Autodesk Inventor part; units mm, degrees
(part 2 of 2)
sketch "Sketch2" plane through (-23.709139, -13.853617, 14.249199) normal (0, 0.9970894, 0.0762418) x (1, 0, 0)
  line L0 (0, 0.624975) -> (-23.2, 0.624975)
  line L1 (0, 0.624975) -> (-23.2, 0.624975)
  line L2 (-23.2, 0.624975) -> (-23.2, 65.920816)
  line L3 (-23.2, 65.920816) -> (0, 65.920816)
  line L4 (0, 65.920816) -> (0, 0.624975)
  circle A0 centre (-9.208398, 23.610194) radius 8 construction
  circle A1 centre (-13, 35.626174) radius 9.6 construction
  circle A2 centre (-9.208398, 23.610194) radius 8.4
  circle A3 centre (-13, 35.626174) radius 10
  circle A4 centre (-9.208398, 23.610194) radius 1.25
  arc A5 (-17.179273, 22.928177) -> (-16.018307, 22.666389) centre (-15.506202, 27.642647) ccw
  arc A6 (-16.018307, 22.666389) -> (-15.959579, 22.311279) centre (-9.208398, 23.610194) ccw
  arc A7 (-15.959579, 22.311279) -> (-16.974447, 21.689654) centre (-13.872622, 17.764852) ccw
  arc A8 (-16.974447, 21.689654) -> (-16.863291, 21.285842) centre (-9.208398, 23.610194) ccw
  arc A9 (-16.863291, 21.285842) -> (-15.673266, 21.271154) centre (-16.206974, 26.245141) ccw
  arc A10 (-15.673266, 21.271154) -> (-15.54199, 20.936014) centre (-9.208398, 23.610194) ccw
  arc A11 (-15.54199, 20.936014) -> (-16.405438, 20.11697) centre (-12.555382, 16.92284) ccw
  arc A12 (-16.405438, 20.11697) -> (-16.212753, 19.745093) centre (-9.208398, 23.610194) ccw
  arc A13 (-16.212753, 19.745093) -> (-15.045679, 19.978146) centre (-16.601875, 24.732476) ccw
  arc A14 (-15.045679, 19.978146) -> (-14.847592, 19.677624) centre (-9.208398, 23.610194) ccw
  arc A15 (-14.847592, 19.677624) -> (-15.521883, 18.696957) centre (-11.091863, 16.373097) ccw
  arc A16 (-15.521883, 18.696957) -> (-15.256092, 18.373268) centre (-9.208398, 23.610194) ccw
  arc A17 (-15.256092, 18.373268) -> (-14.162975, 18.843876) centre (-16.673645, 23.170761) ccw
  arc A18 (-14.162975, 18.843876) -> (-13.906735, 18.591106) centre (-9.208398, 23.610194) ccw
  arc A19 (-13.906735, 18.591106) -> (-14.362399, 17.491675) centre (-9.546028, 16.139651) ccw
  arc A20 (-14.362399, 17.491675) -> (-14.035117, 17.230321) centre (-9.208398, 23.610194) ccw
  arc A21 (-14.035117, 17.230321) -> (-13.063732, 17.917917) centre (-16.419148, 21.628251) ccw
  arc A22 (-13.063732, 17.917917) -> (-12.760538, 17.723945) centre (-9.208398, 23.610194) ccw
  arc A23 (-12.760538, 17.723945) -> (-12.97766, 16.553803) centre (-7.985437, 16.232703) ccw
  arc A24 (-12.97766, 16.553803) -> (-12.603191, 16.366205) centre (-9.208398, 23.610194) ccw
  arc A25 (-12.603191, 16.366205) -> (-11.795993, 17.240738) centre (-15.849507, 20.172362) ccw
  arc A26 (-11.795993, 17.240738) -> (-11.459095, 17.114043) centre (-9.208398, 23.610194) ccw
  arc A27 (-11.459095, 17.114043) -> (-11.428186, 15.924328) centre (-6.478294, 16.648187) ccw
  arc A28 (-11.428186, 15.924328) -> (-11.022897, 15.818687) centre (-9.208398, 23.610194) ccw
  arc A29 (-11.022897, 15.818687) -> (-10.415163, 16.841935) centre (-14.989617, 18.866723) ccw
  arc A30 (-10.415163, 16.841935) -> (-10.059286, 16.788053) centre (-9.208398, 23.610194) ccw
  arc A31 (-10.059286, 16.788053) -> (-9.781697, 15.630763) centre (-5.090471, 17.367944) ccw
  arc A32 (-9.781697, 15.630763) -> (-9.3633, 15.611694) centre (-9.208398, 23.610194) ccw
  arc A33 (-9.3633, 15.611694) -> (-8.981592, 16.738937) centre (-13.87706, 17.768396) ccw
  arc A34 (-8.981592, 16.738937) -> (-8.622289, 16.760224) centre (-9.208398, 23.610194) ccw
  arc A35 (-8.622289, 16.760224) -> (-8.110152, 15.685937) centre (-3.882621, 18.360517) ccw
  arc A36 (-8.110152, 15.685937) -> (-7.696933, 15.754275) centre (-9.208398, 23.610194) ccw
  arc A37 (-7.696933, 15.754275) -> (-7.557934, 16.936246) centre (-12.560461, 16.925384) ccw
  arc A38 (-7.557934, 16.936246) -> (-7.210908, 17.031771) centre (-9.208398, 23.610194) ccw
  arc A39 (-7.210908, 17.031771) -> (-6.486605, 16.087439) centre (-2.907532, 19.582526) ccw
  arc A40 (-6.486605, 16.087439) -> (-6.096625, 16.240197) centre (-9.208398, 23.610194) ccw
  arc A41 (-6.096625, 16.240197) -> (-6.206408, 17.425238) centre (-11.09736, 16.37453) ccw
  arc A42 (-6.206408, 17.425238) -> (-5.886827, 17.590827) centre (-9.208398, 23.610194) ccw
  arc A43 (-5.886827, 17.590827) -> (-4.982014, 16.817722) centre (-2.207822, 20.980564) ccw
  arc A44 (-4.982014, 16.817722) -> (-4.632316, 17.048223) centre (-9.208398, 23.610194) ccw
  arc A45 (-4.632316, 17.048223) -> (-4.986084, 18.184543) centre (-9.551702, 16.139909) ccw
  arc A46 (-4.986084, 18.184543) -> (-4.707914, 18.412958) centre (-9.208398, 23.610194) ccw
  arc A47 (-4.707914, 18.412958) -> (-3.662136, 17.844868) centre (-1.81407, 22.493529) ccw
  arc A48 (-3.662136, 17.844868) -> (-3.368003, 18.143039) centre (-9.208398, 23.610194) ccw
  arc A49 (-3.368003, 18.143039) -> (-3.950295, 19.180975) centre (-7.991041, 16.231776) ccw
  arc A50 (-3.950295, 19.180975) -> (-3.725694, 19.462233) centre (-9.208398, 23.610194) ccw
  arc A51 (-3.725694, 19.462233) -> (-2.584657, 19.123987) centre (-1.743487, 24.055298) ccw
  arc A52 (-2.584657, 19.123987) -> (-2.358945, 19.476795) centre (-9.208398, 23.610194) ccw
  arc A53 (-2.358945, 19.476795) -> (-3.144311, 20.370985) centre (-6.483583, 16.646115) ccw
  arc A54 (-3.144311, 20.370985) -> (-2.983095, 20.692794) centre (-9.208398, 23.610194) ccw
  arc A55 (-2.983095, 20.692794) -> (-1.796667, 20.599175) centre (-1.999155, 25.597614) ccw
  arc A56 (-1.796667, 20.599175) -> (-1.649239, 20.991201) centre (-9.208398, 23.610194) ccw
  arc A57 (-1.649239, 20.991201) -> (-2.603356, 21.702564) centre (-5.095213, 17.364818) ccw
  arc A58 (-2.603356, 21.702564) -> (-2.512571, 22.05086) centre (-9.208398, 23.610194) ccw
  arc A59 (-2.512571, 22.05086) -> (-1.332604, 22.205958) centre (-2.569902, 27.05307) ccw
  arc A60 (-1.332604, 22.205958) -> (-1.269906, 22.62007) centre (-9.208398, 23.610194) ccw
  arc A61 (-1.269906, 22.62007) -> (-2.351074, 23.117516) centre (-3.886609, 18.356473) ccw
  arc A62 (-2.351074, 23.117516) -> (-2.334687, 23.477076) centre (-9.208398, 23.610194) ccw
  arc A63 (-2.334687, 23.477076) -> (-1.212752, 23.874114) centre (-3.430783, 28.358056) ccw
  arc A64 (-1.212752, 23.874114) -> (-1.237523, 24.292212) centre (-9.208398, 23.610194) ccw
  arc A65 (-1.237523, 24.292212) -> (-2.398489, 24.554) centre (-2.910593, 19.577742) ccw
  arc A66 (-2.398489, 24.554) -> (-2.457217, 24.909109) centre (-9.208398, 23.610194) ccw
  arc A67 (-2.457217, 24.909109) -> (-1.442348, 25.530735) centre (-4.544174, 29.455537) ccw
  arc A68 (-1.442348, 25.530735) -> (-1.553505, 25.934546) centre (-9.208398, 23.610194) ccw
  arc A69 (-1.553505, 25.934546) -> (-2.74353, 25.949235) centre (-2.209821, 20.975248) ccw
  arc A70 (-2.74353, 25.949235) -> (-2.874806, 26.284374) centre (-9.208398, 23.610194) ccw
  arc A71 (-2.874806, 26.284374) -> (-2.011358, 27.103419) centre (-5.861413, 30.297549) ccw
  arc A72 (-2.011358, 27.103419) -> (-2.204043, 27.475295) centre (-9.208398, 23.610194) ccw
  arc A73 (-2.204043, 27.475295) -> (-3.371117, 27.242243) centre (-1.814921, 22.487913) ccw
  arc A74 (-3.371117, 27.242243) -> (-3.569203, 27.542765) centre (-9.208398, 23.610194) ccw
  arc A75 (-3.569203, 27.542765) -> (-2.894913, 28.523432) centre (-7.324932, 30.847292) ccw
  arc A76 (-2.894913, 28.523432) -> (-3.160704, 28.847121) centre (-9.208398, 23.610194) ccw
  arc A77 (-3.160704, 28.847121) -> (-4.253821, 28.376513) centre (-1.743151, 24.049628) ccw
  arc A78 (-4.253821, 28.376513) -> (-4.510061, 28.629283) centre (-9.208398, 23.610194) ccw
  arc A79 (-4.510061, 28.629283) -> (-4.054397, 29.728714) centre (-8.870768, 31.080738) ccw
  arc A80 (-4.054397, 29.728714) -> (-4.381679, 29.990068) centre (-9.208398, 23.610194) ccw
  arc A81 (-4.381679, 29.990068) -> (-5.353064, 29.302472) centre (-1.997648, 25.592138) ccw
  arc A82 (-5.353064, 29.302472) -> (-5.656258, 29.496443) centre (-9.208398, 23.610194) ccw
  arc A83 (-5.656258, 29.496443) -> (-5.439136, 30.666586) centre (-10.431359, 30.987686) ccw
  arc A84 (-5.439136, 30.666586) -> (-5.813605, 30.854184) centre (-9.208398, 23.610194) ccw
  arc A85 (-5.813605, 30.854184) -> (-6.620803, 29.979651) centre (-2.567289, 27.048027) ccw
  arc A86 (-6.620803, 29.979651) -> (-6.957701, 30.106346) centre (-9.208398, 23.610194) ccw
  arc A87 (-6.957701, 30.106346) -> (-6.98861, 31.296061) centre (-11.938501, 30.572202) ccw
  arc A88 (-6.98861, 31.296061) -> (-7.393899, 31.401702) centre (-9.208398, 23.610194) ccw
  arc A89 (-7.393899, 31.401702) -> (-8.001633, 30.378454) centre (-3.427179, 28.353666) ccw
  arc A90 (-8.001633, 30.378454) -> (-8.35751, 30.432336) centre (-9.208398, 23.610194) ccw
  arc A91 (-8.35751, 30.432336) -> (-8.635099, 31.589626) centre (-13.326325, 29.852445) ccw
  arc A92 (-8.635099, 31.589626) -> (-9.053496, 31.608695) centre (-9.208398, 23.610194) ccw
  arc A93 (-9.053496, 31.608695) -> (-9.435204, 30.481452) centre (-4.539735, 29.451993) ccw
  arc A94 (-9.435204, 30.481452) -> (-9.794507, 30.460165) centre (-9.208398, 23.610194) ccw
  arc A95 (-9.794507, 30.460165) -> (-10.306644, 31.534452) centre (-14.534175, 28.859872) ccw
  arc A96 (-10.306644, 31.534452) -> (-10.719863, 31.466114) centre (-9.208398, 23.610194) ccw
  arc A97 (-10.719863, 31.466114) -> (-10.858862, 30.284143) centre (-5.856335, 30.295005) ccw
  arc A98 (-10.858862, 30.284143) -> (-11.205888, 30.188618) centre (-9.208398, 23.610194) ccw
  arc A99 (-11.205888, 30.188618) -> (-11.930191, 31.13295) centre (-15.509264, 27.637863) ccw
  arc A100 (-11.930191, 31.13295) -> (-12.320171, 30.980192) centre (-9.208398, 23.610194) ccw
  arc A101 (-12.320171, 30.980192) -> (-12.210388, 29.795151) centre (-7.319436, 30.845859) ccw
  arc A102 (-12.210388, 29.795151) -> (-12.529969, 29.629562) centre (-9.208398, 23.610194) ccw
  arc A103 (-12.529969, 29.629562) -> (-13.434782, 30.402667) centre (-16.208974, 26.239825) ccw
  arc A104 (-13.434782, 30.402667) -> (-13.78448, 30.172166) centre (-9.208398, 23.610194) ccw
  arc A105 (-13.78448, 30.172166) -> (-13.430712, 29.035846) centre (-8.865094, 31.08048) ccw
  arc A106 (-13.430712, 29.035846) -> (-13.708882, 28.807431) centre (-9.208398, 23.610194) ccw
  arc A107 (-13.708882, 28.807431) -> (-14.754659, 29.37552) centre (-16.602725, 24.726859) ccw
  arc A108 (-14.754659, 29.37552) -> (-15.048792, 29.07735) centre (-9.208398, 23.610194) ccw
  arc A109 (-15.048792, 29.07735) -> (-14.4665, 28.039414) centre (-10.425755, 30.988613) ccw
  arc A110 (-14.4665, 28.039414) -> (-14.691102, 27.758156) centre (-9.208398, 23.610194) ccw
  arc A111 (-14.691102, 27.758156) -> (-15.832139, 28.096402) centre (-16.673309, 23.165091) ccw
  arc A112 (-15.832139, 28.096402) -> (-16.057851, 27.743594) centre (-9.208398, 23.610194) ccw
  arc A113 (-16.057851, 27.743594) -> (-15.272485, 26.849404) centre (-11.933213, 30.574274) ccw
  arc A114 (-15.272485, 26.849404) -> (-15.433701, 26.527595) centre (-9.208398, 23.610194) ccw
  arc A115 (-15.433701, 26.527595) -> (-16.620129, 26.621214) centre (-16.417641, 21.622775) ccw
  arc A116 (-16.620129, 26.621214) -> (-16.767556, 26.229187) centre (-9.208398, 23.610194) ccw
  arc A117 (-16.767556, 26.229187) -> (-15.813439, 25.517825) centre (-13.321582, 29.855571) ccw
  arc A118 (-15.813439, 25.517825) -> (-15.904225, 25.169529) centre (-9.208398, 23.610194) ccw
  arc A119 (-15.904225, 25.169529) -> (-17.084191, 25.01443) centre (-15.846894, 20.167319) ccw
  arc A120 (-17.084191, 25.01443) -> (-17.14689, 24.600319) centre (-9.208398, 23.610194) ccw
  arc A121 (-17.14689, 24.600319) -> (-16.065722, 24.102873) centre (-14.530186, 28.863916) ccw
  arc A122 (-16.065722, 24.102873) -> (-16.082109, 23.743313) centre (-9.208398, 23.610194) ccw
  arc A123 (-16.082109, 23.743313) -> (-17.204043, 23.346275) centre (-14.986013, 18.862333) ccw
  arc A124 (-17.204043, 23.346275) -> (-17.179273, 22.928177) centre (-9.208398, 23.610194) ccw
  arc A125 (-20.63224, 38.75849) -> (-22.059739, 38.801252) centre (-21.52446, 32.822118) ccw
  arc A126 (-22.059739, 38.801252) -> (-22.213494, 38.322751) centre (-13, 35.626174) ccw
  arc A127 (-22.213494, 38.322751) -> (-21.028277, 37.525981) centre (-18.295517, 42.87094) ccw
  arc A128 (-21.028277, 37.525981) -> (-21.116703, 37.10321) centre (-13, 35.626174) ccw
  arc A129 (-21.116703, 37.10321) -> (-22.521898, 36.848243) centre (-20.755184, 31.111058) ccw
  arc A130 (-22.521898, 36.848243) -> (-22.572807, 36.348231) centre (-13, 35.626174) ccw
  arc A131 (-22.572807, 36.348231) -> (-21.247832, 35.815293) centre (-19.686069, 41.611625) ccw
  arc A132 (-21.247832, 35.815293) -> (-21.246426, 35.383375) centre (-13, 35.626174) ccw
  arc A133 (-21.246426, 35.383375) -> (-22.567904, 34.841824) centre (-19.64697, 29.597331) ccw
  arc A134 (-22.567904, 34.841824) -> (-22.513742, 34.342154) centre (-13, 35.626174) ccw
  arc A135 (-22.513742, 34.342154) -> (-21.106917, 34.096339) centre (-20.784408, 40.090717) ccw
  arc A136 (-21.106917, 34.096339) -> (-21.015742, 33.674153) centre (-13, 35.626174) ccw
  arc A137 (-21.015742, 33.674153) -> (-22.195747, 32.869685) centre (-18.248251, 28.347093) ccw
  arc A138 (-22.195747, 32.869685) -> (-22.038882, 32.392195) centre (-13, 35.626174) ccw
  arc A139 (-22.038882, 32.392195) -> (-20.611691, 32.444247) centre (-21.54253, 38.374686) ccw
  arc A140 (-20.611691, 32.444247) -> (-20.434731, 32.050243) centre (-13, 35.626174) ccw
  arc A141 (-20.434731, 32.050243) -> (-21.421692, 31.018018) centre (-16.620158, 27.414986) ccw
  arc A142 (-21.421692, 31.018018) -> (-21.168978, 30.583576) centre (-13, 35.626174) ccw
  arc A143 (-21.168978, 30.583576) -> (-19.783798, 30.93122) centre (-21.927304, 36.538533) ccw
  arc A144 (-19.783798, 30.93122) -> (-19.528786, 30.582618) centre (-13, 35.626174) ccw
  arc A145 (-19.528786, 30.582618) -> (-20.279568, 29.367749) centre (-14.833847, 26.841747) ccw
  arc A146 (-20.279568, 29.367749) -> (-19.942051, 28.995342) centre (-13, 35.626174) ccw
  arc A147 (-19.942051, 28.995342) -> (-18.65942, 29.623385) centre (-21.921911, 34.662505) ccw
  arc A148 (-18.65942, 29.623385) -> (-18.337502, 29.335421) centre (-13, 35.626174) ccw
  arc A149 (-18.337502, 29.335421) -> (-18.819293, 27.991003) centre (-12.967388, 26.652429) ccw
  arc A150 (-18.819293, 27.991003) -> (-18.411724, 27.696908) centre (-13, 35.626174) ccw
  arc A151 (-18.411724, 27.696908) -> (-17.287698, 28.577901) centre (-21.526587, 32.828594) ccw
  arc A152 (-17.287698, 28.577901) -> (-16.912944, 28.36316) centre (-13, 35.626174) ccw
  arc A153 (-16.912944, 28.36316) -> (-17.104686, 26.947951) centre (-11.102354, 26.855308) ccw
  arc A154 (-17.104686, 26.947951) -> (-16.644878, 26.745021) centre (-13, 35.626174) ccw
  arc A155 (-16.644878, 26.745021) -> (-15.728583, 27.84046) centre (-20.758611, 31.11695) ccw
  arc A156 (-15.728583, 27.84046) -> (-15.317371, 27.708327) centre (-13, 35.626174) ccw
  arc A157 (-15.317371, 27.708327) -> (-15.210685, 26.284178) centre (-9.320257, 27.441515) ccw
  arc A158 (-15.210685, 26.284178) -> (-14.718733, 26.181283) centre (-13, 35.626174) ccw
  arc A159 (-14.718733, 26.181283) -> (-14.050216, 27.443292) centre (-19.651547, 29.602382) ccw
  arc A160 (-14.050216, 27.443292) -> (-13.620518, 27.399543) centre (-13, 35.626174) ccw
  arc A161 (-13.620518, 27.399543) -> (-13.220066, 26.028696) centre (-7.698982, 28.385431) ccw
  arc A162 (-13.220066, 26.028696) -> (-12.717471, 26.030332) centre (-13, 35.626174) ccw
  arc A163 (-12.717471, 26.030332) -> (-12.32595, 27.403756) centre (-18.253778, 28.351081) ccw
  arc A164 (-12.32595, 27.403756) -> (-11.896546, 27.450301) centre (-13, 35.626174) ccw
  arc A165 (-11.896546, 27.450301) -> (-11.219829, 26.19267) centre (-6.309387, 29.645802) ccw
  arc A166 (-11.219829, 26.19267) -> (-10.728557, 26.298765) centre (-13, 35.626174) ccw
  arc A167 (-10.728557, 26.298765) -> (-10.631143, 27.723578) centre (-16.626394, 27.417738) ccw
  arc A168 (-10.631143, 27.723578) -> (-10.220799, 27.858385) centre (-13, 35.626174) ccw
  arc A169 (-10.220799, 27.858385) -> (-9.297395, 26.768933) centre (-5.212203, 31.167544) ccw
  arc A170 (-9.297395, 26.768933) -> (-8.838917, 26.974851) centre (-13, 35.626174) ccw
  arc A171 (-8.838917, 26.974851) -> (-9.039866, 28.388782) centre (-14.840518, 26.843142) ccw
  arc A172 (-9.039866, 28.388782) -> (-8.666517, 28.605958) centre (-13, 35.626174) ccw
  arc A173 (-8.666517, 28.605958) -> (-7.536781, 27.7323) centre (-4.455384, 32.88415) ccw
  arc A174 (-7.536781, 27.7323) -> (-7.131135, 28.029041) centre (-13, 35.626174) ccw
  arc A175 (-7.131135, 28.029041) -> (-7.621666, 29.370294) centre (-12.974204, 26.652407) ccw
  arc A176 (-7.621666, 29.370294) -> (-7.301629, 29.660348) centre (-13, 35.626174) ccw
  arc A177 (-7.301629, 29.660348) -> (-6.014937, 29.040667) centre (-4.072006, 34.720595) ccw
  arc A178 (-6.014937, 29.040667) -> (-5.679851, 29.415262) centre (-13, 35.626174) ccw
  arc A179 (-5.679851, 29.415262) -> (-6.438525, 30.625219) centre (-11.109017, 26.853869) ccw
  arc A180 (-6.438525, 30.625219) -> (-6.185788, 30.975474) centre (-13, 35.626174) ccw
  arc A181 (-6.185788, 30.975474) -> (-4.798374, 30.636852) centre (-4.078824, 36.596619) ccw
  arc A182 (-4.798374, 30.636852) -> (-4.548493, 31.07293) centre (-13, 35.626174) ccw
  arc A183 (-4.548493, 31.07293) -> (-5.542152, 32.098709) centre (-9.326474, 27.438722) ccw
  arc A184 (-5.542152, 32.098709) -> (-5.36776, 32.493857) centre (-13, 35.626174) ccw
  arc A185 (-5.36776, 32.493857) -> (-3.940261, 32.451095) centre (-4.47554, 38.430229) ccw
  arc A186 (-3.940261, 32.451095) -> (-3.786506, 32.929596) centre (-13, 35.626174) ccw
  arc A187 (-3.786506, 32.929596) -> (-4.971723, 33.726366) centre (-7.704483, 28.381407) ccw
  arc A188 (-4.971723, 33.726366) -> (-4.883297, 34.149138) centre (-13, 35.626174) ccw
  arc A189 (-4.883297, 34.149138) -> (-3.478102, 34.404104) centre (-5.244816, 40.141289) ccw
  arc A190 (-3.478102, 34.404104) -> (-3.427193, 34.904116) centre (-13, 35.626174) ccw
  arc A191 (-3.427193, 34.904116) -> (-4.752168, 35.437054) centre (-6.313931, 29.640722) ccw
  arc A192 (-4.752168, 35.437054) -> (-4.753574, 35.868972) centre (-13, 35.626174) ccw
  arc A193 (-4.753574, 35.868972) -> (-3.432096, 36.410523) centre (-6.35303, 41.655016) ccw
  arc A194 (-3.432096, 36.410523) -> (-3.486258, 36.910193) centre (-13, 35.626174) ccw
  arc A195 (-3.486258, 36.910193) -> (-4.893083, 37.156008) centre (-5.215592, 31.161631) ccw
  arc A196 (-4.893083, 37.156008) -> (-4.984258, 37.578194) centre (-13, 35.626174) ccw
  arc A197 (-4.984258, 37.578194) -> (-3.804253, 38.382662) centre (-7.751749, 42.905254) ccw
  arc A198 (-3.804253, 38.382662) -> (-3.961118, 38.860153) centre (-13, 35.626174) ccw
  arc A199 (-3.961118, 38.860153) -> (-5.388309, 38.8081) centre (-4.45747, 32.877661) ccw
  arc A200 (-5.388309, 38.8081) -> (-5.565269, 39.202104) centre (-13, 35.626174) ccw
  arc A201 (-5.565269, 39.202104) -> (-4.578308, 40.234329) centre (-9.379842, 43.837361) ccw
  arc A202 (-4.578308, 40.234329) -> (-4.831022, 40.668771) centre (-13, 35.626174) ccw
  arc A203 (-4.831022, 40.668771) -> (-6.216202, 40.321127) centre (-4.072696, 34.713814) ccw
  arc A204 (-6.216202, 40.321127) -> (-6.471214, 40.669729) centre (-13, 35.626174) ccw
  arc A205 (-6.471214, 40.669729) -> (-5.720432, 41.884598) centre (-11.166153, 44.4106) ccw
  arc A206 (-5.720432, 41.884598) -> (-6.057949, 42.257005) centre (-13, 35.626174) ccw
  arc A207 (-6.057949, 42.257005) -> (-7.34058, 41.628962) centre (-4.078089, 36.589842) ccw
  arc A208 (-7.34058, 41.628962) -> (-7.662498, 41.916926) centre (-13, 35.626174) ccw
  arc A209 (-7.662498, 41.916926) -> (-7.180707, 43.261344) centre (-13.032612, 44.599918) ccw
  arc A210 (-7.180707, 43.261344) -> (-7.588276, 43.555439) centre (-13, 35.626174) ccw
  arc A211 (-7.588276, 43.555439) -> (-8.712302, 42.674446) centre (-4.473413, 38.423753) ccw
  arc A212 (-8.712302, 42.674446) -> (-9.087056, 42.889187) centre (-13, 35.626174) ccw
  arc A213 (-9.087056, 42.889187) -> (-8.895314, 44.304396) centre (-14.897646, 44.397039) ccw
  arc A214 (-8.895314, 44.304396) -> (-9.355122, 44.507326) centre (-13, 35.626174) ccw
  arc A215 (-9.355122, 44.507326) -> (-10.271417, 43.411887) centre (-5.241389, 40.135397) ccw
  arc A216 (-10.271417, 43.411887) -> (-10.682629, 43.54402) centre (-13, 35.626174) ccw
  arc A217 (-10.682629, 43.54402) -> (-10.789315, 44.968169) centre (-16.679743, 43.810832) ccw
  arc A218 (-10.789315, 44.968169) -> (-11.281267, 45.071064) centre (-13, 35.626174) ccw
  arc A219 (-11.281267, 45.071064) -> (-11.949784, 43.809055) centre (-6.348453, 41.649966) ccw
  arc A220 (-11.949784, 43.809055) -> (-12.379482, 43.852804) centre (-13, 35.626174) ccw
  arc A221 (-12.379482, 43.852804) -> (-12.779934, 45.223651) centre (-18.301018, 42.866916) ccw
  arc A222 (-12.779934, 45.223651) -> (-13.282529, 45.222015) centre (-13, 35.626174) ccw
  arc A223 (-13.282529, 45.222015) -> (-13.67405, 43.848591) centre (-7.746222, 42.901266) ccw
  arc A224 (-13.67405, 43.848591) -> (-14.103454, 43.802046) centre (-13, 35.626174) ccw
  arc A225 (-14.103454, 43.802046) -> (-14.780171, 45.059677) centre (-19.690613, 41.606545) ccw
  arc A226 (-14.780171, 45.059677) -> (-15.271443, 44.953582) centre (-13, 35.626174) ccw
  arc A227 (-15.271443, 44.953582) -> (-15.368857, 43.528769) centre (-9.373606, 43.834609) ccw
  arc A228 (-15.368857, 43.528769) -> (-15.779201, 43.393962) centre (-13, 35.626174) ccw
  arc A229 (-15.779201, 43.393962) -> (-16.702605, 44.483414) centre (-20.787797, 40.084803) ccw
  arc A230 (-16.702605, 44.483414) -> (-17.161083, 44.277496) centre (-13, 35.626174) ccw
  arc A231 (-17.161083, 44.277496) -> (-16.960134, 42.863565) centre (-11.159482, 44.409205) ccw
  arc A232 (-16.960134, 42.863565) -> (-17.333483, 42.646389) centre (-13, 35.626174) ccw
  arc A233 (-17.333483, 42.646389) -> (-18.463219, 43.520047) centre (-21.544616, 38.368197) ccw
  arc A234 (-18.463219, 43.520047) -> (-18.868865, 43.223306) centre (-13, 35.626174) ccw
  arc A235 (-18.868865, 43.223306) -> (-18.378334, 41.882053) centre (-13.025796, 44.59994) ccw
  arc A236 (-18.378334, 41.882053) -> (-18.698371, 41.591999) centre (-13, 35.626174) ccw
  arc A237 (-18.698371, 41.591999) -> (-19.985063, 42.21168) centre (-21.927994, 36.531752) ccw
  arc A238 (-19.985063, 42.21168) -> (-20.320149, 41.837085) centre (-13, 35.626174) ccw
  arc A239 (-20.320149, 41.837085) -> (-19.561475, 40.627128) centre (-14.890983, 44.398478) ccw
  arc A240 (-19.561475, 40.627128) -> (-19.814212, 40.276874) centre (-13, 35.626174) ccw
  arc A241 (-19.814212, 40.276874) -> (-21.201626, 40.615495) centre (-21.921176, 34.655728) ccw
  arc A242 (-21.201626, 40.615495) -> (-21.451507, 40.179417) centre (-13, 35.626174) ccw
  arc A243 (-21.451507, 40.179417) -> (-20.457848, 39.153638) centre (-16.673526, 43.813625) ccw
  arc A244 (-20.457848, 39.153638) -> (-20.63224, 38.75849) centre (-13, 35.626174) ccw
  circle A245 centre (-14.5, 55.920816) radius 14.5
  circle A246 centre (-14.5, 55.920816) radius 13.85
  circle A247 centre (-14.5, 15.124975) radius 14.5
  circle A248 centre (-14.5, 15.124975) radius 13.85
  circle A249 centre (-14.5, 15.124975) radius 5
  circle A250 centre (-13, 35.626174) radius 5
  point P0 (23.709139, 15.26395)
  point P1 (-7.76131, 27.58154)
  point P2 (-4.410688, 30.505264)
  point P3 (-17.094606, 26.502896)
  point P4 (-23.2, 0.624975)
  point P5 (-9.500816, 15.215286)
  point P6 (-16.618436, 19.654018)
  dimension "d14" = 0.4
  dimension "d15" = 0.4
  dimension "d16" = 0.2
  dimension "d128" = 4.5
  constraints: 8 end point, 3 centre point, 2 coincident, 2 parallel, 2 point on circle, 1 horizontal, 1 perpendicular, 4 other
  measures "d15" radial gap between concentric circles of A1 A3
  measures "d16" distance edge to line of A3 L2
  measures "d128" distance edge to line of A245 L3
extrude "Extrusion5" add sketch "Sketch2" along normal blind 3.7 contours L0 A247 L4 | L0 L2 A247 | A247 L2 A248 A2 | A247 A2 A3 A245 L4 | A245 L3 L4 | A245 A3 A246 L3 | L2 A248 A3 A2 A249 | A247 A3 A248 L2 | L2 A245 A3 A247 | L2 A246 A3 A245 | A246 A3 L2 L3
ref_plane "Work Plane7" through (-38.132644, -18.241727, -0.502049) normal (0, 0.9970894, 0.0762418) x (-0.6440904, -0.0583212, 0.7627229)
sketch "Sketch12" plane through (-38.132644, -18.241727, -0.502049) normal (0, 0.9970894, 0.0762418) x (-0.6440904, -0.0583212, 0.7627229)
  circle A0 centre (-10.439114, -1.949408) radius 4.2 construction
  circle A1 centre (-10.439114, -1.949408) radius 4.6
  circle A2 centre (-10.439114, -1.949408) radius 1.25
  arc A3 (-14.254475, -0.193555) -> (-13.161478, -1.106062) centre (-11.37806, 2.140957) ccw
  arc A4 (-13.161478, -1.106062) -> (-13.248266, -1.468616) centre (-10.439114, -1.949408) ccw
  arc A5 (-13.248266, -1.468616) -> (-14.635984, -1.787287) centre (-13.128458, -5.171231) ccw
  arc A6 (-14.635984, -1.787287) -> (-14.62124, -2.336476) centre (-10.439114, -1.949408) ccw
  arc A7 (-14.62124, -2.336476) -> (-13.218424, -2.580231) centre (-13.297448, 1.123479) ccw
  arc A8 (-13.218424, -2.580231) -> (-13.112307, -2.937607) centre (-10.439114, -1.949408) ccw
  arc A9 (-13.112307, -2.937607) -> (-14.15477, -3.907442) centre (-11.157243, -6.084261) ccw
  arc A10 (-14.15477, -3.907442) -> (-13.867408, -4.375682) centre (-10.439114, -1.949408) ccw
  arc A11 (-13.867408, -4.375682) -> (-12.530656, -3.885372) centre (-14.450948, -0.717377) ccw
  arc A12 (-12.530656, -3.885372) -> (-12.260068, -4.14181) centre (-10.439114, -1.949408) ccw
  arc A13 (-12.260068, -4.14181) -> (-12.67795, -5.502944) centre (-8.993605, -5.88936) ccw
  arc A14 (-12.67795, -5.502944) -> (-12.194967, -5.76477) centre (-10.439114, -1.949408) ccw
  arc A15 (-12.194967, -5.76477) -> (-11.282461, -4.671773) centre (-14.52948, -2.888355) ccw
  arc A16 (-11.282461, -4.671773) -> (-10.919906, -4.758561) centre (-10.439114, -1.949408) ccw
  arc A17 (-10.919906, -4.758561) -> (-10.601235, -6.146278) centre (-7.217291, -4.638753) ccw
  arc A18 (-10.601235, -6.146278) -> (-10.052047, -6.131535) centre (-10.439114, -1.949408) ccw
  arc A19 (-10.052047, -6.131535) -> (-9.808291, -4.728718) centre (-13.512001, -4.807743) ccw
  arc A20 (-9.808291, -4.728718) -> (-9.450916, -4.622602) centre (-10.439114, -1.949408) ccw
  arc A21 (-9.450916, -4.622602) -> (-8.48108, -5.665065) centre (-6.304261, -2.667537) ccw
  arc A22 (-8.48108, -5.665065) -> (-8.012841, -5.377702) centre (-10.439114, -1.949408) ccw
  arc A23 (-8.012841, -5.377702) -> (-8.503151, -4.04095) centre (-11.671145, -5.961243) ccw
  arc A24 (-8.503151, -4.04095) -> (-8.246712, -3.770363) centre (-10.439114, -1.949408) ccw
  arc A25 (-8.246712, -3.770363) -> (-6.885578, -4.188245) centre (-6.499162, -0.5039) ccw
  arc A26 (-6.885578, -4.188245) -> (-6.623753, -3.705262) centre (-10.439114, -1.949408) ccw
  arc A27 (-6.623753, -3.705262) -> (-7.71675, -2.792755) centre (-9.500167, -6.039774) ccw
  arc A28 (-7.71675, -2.792755) -> (-7.629961, -2.430201) centre (-10.439114, -1.949408) ccw
  arc A29 (-7.629961, -2.430201) -> (-6.242244, -2.11153) centre (-7.74977, 1.272414) ccw
  arc A30 (-6.242244, -2.11153) -> (-6.256988, -1.562341) centre (-10.439114, -1.949408) ccw
  arc A31 (-6.256988, -1.562341) -> (-7.659804, -1.318586) centre (-7.580779, -5.022296) ccw
  arc A32 (-7.659804, -1.318586) -> (-7.76592, -0.96121) centre (-10.439114, -1.949408) ccw
  arc A33 (-7.76592, -0.96121) -> (-6.723457, 0.008625) centre (-9.720985, 2.185444) ccw
  arc A34 (-6.723457, 0.008625) -> (-7.01082, 0.476865) centre (-10.439114, -1.949408) ccw
  arc A35 (-7.01082, 0.476865) -> (-8.347572, -0.013445) centre (-6.42728, -3.18144) ccw
  arc A36 (-8.347572, -0.013445) -> (-8.618159, 0.242993) centre (-10.439114, -1.949408) ccw
  arc A37 (-8.618159, 0.242993) -> (-8.200278, 1.604127) centre (-11.884622, 1.990543) ccw
  arc A38 (-8.200278, 1.604127) -> (-8.683261, 1.865953) centre (-10.439114, -1.949408) ccw
  arc A39 (-8.683261, 1.865953) -> (-9.595767, 0.772956) centre (-6.348748, -1.010462) ccw
  arc A40 (-9.595767, 0.772956) -> (-9.958322, 0.859744) centre (-10.439114, -1.949408) ccw
  arc A41 (-9.958322, 0.859744) -> (-10.276993, 2.247461) centre (-13.660937, 0.739936) ccw
  arc A42 (-10.276993, 2.247461) -> (-10.826181, 2.232718) centre (-10.439114, -1.949408) ccw
  arc A43 (-10.826181, 2.232718) -> (-11.069936, 0.829901) centre (-7.366226, 0.908926) ccw
  arc A44 (-11.069936, 0.829901) -> (-11.427312, 0.723785) centre (-10.439114, -1.949408) ccw
  arc A45 (-11.427312, 0.723785) -> (-12.397148, 1.766248) centre (-14.573966, -1.23128) ccw
  arc A46 (-12.397148, 1.766248) -> (-12.865387, 1.478885) centre (-10.439114, -1.949408) ccw
  arc A47 (-12.865387, 1.478885) -> (-12.375077, 0.142133) centre (-9.207082, 2.062426) ccw
  arc A48 (-12.375077, 0.142133) -> (-12.631515, -0.128454) centre (-10.439114, -1.949408) ccw
  arc A49 (-12.631515, -0.128454) -> (-13.992649, 0.289428) centre (-14.379065, -3.394917) ccw
  arc A50 (-13.992649, 0.289428) -> (-14.254475, -0.193555) centre (-10.439114, -1.949408) ccw
  point P0 (-25.241823, 28.596177)
  point P1 (-6.334554, -1.059132)
  dimension "d110" = 0.4
  constraints: 2 centre point, 2 point on circle, 1 coincident
  measures "d110" radial gap between concentric circles of A0 A1
extrude "Extrusion9" add sketch "Sketch12" along normal blind 1.5 contours A1 | A2 | A50 A49 A48 A47 A46 A45 A44 A43 A42 A41 A40 A39 A38 A37 A36 A35 A34 A33 A32 A31 A30 A29 A28 A27 A26 A25 A24 A23 A22 A21 A20 A19 A18 A17 A16 A15 A14 A13 A12 A11 A10 A9 A8 A7 A6 A5 A4 A3
sketch "Sketch3" plane through (-23.709139, -10.164386, 14.531294) normal (0, 0.9970894, 0.0762418) x (1, 0, 0)
  line L0 (-1.5, 17.124975) -> (-1.5, 1.124975)
  line L1 (-2.5, 17.124975) -> (-1.5, 17.124975)
  line L2 (-2.5, 1.124975) -> (-2.5, 17.124975)
  line L3 (-2.5, 1.124975) -> (-1.5, 1.124975)
  line L4 (-1.5, 1.124975) -> (-1, 1.124975)
  line L5 (-1, 1.124975) -> (-1, 17.624975)
  line L6 (-1, 17.624975) -> (-2.5, 17.624975)
  line L7 (-2.5, 17.624975) -> (-2.5, 17.124975)
  point P0 (23.709139, 15.26395)
  dimension "d20" = 0.5
  dimension "d21" = 0.5
  constraints: 8 end point, 3 perpendicular, 1 horizontal
  measures "d20" distance between parallel lines of L6 L1
  measures "d21" distance between parallel lines of L5 L0
extrude "Extrusion6" cut sketch "Sketch3" against normal blind 7.1
sketch "Sketch4" plane through (-23.709139, -10.164386, 14.531294) normal (0, 0.9970894, 0.0762418) x (1, 0, 0)
  line L0 (-1.459131, 17.124975) -> (-1.459131, 1.124975)
  line L1 (-2.459131, 17.124975) -> (-1.459131, 17.124975)
  line L2 (-2.459131, 1.124975) -> (-2.459131, 17.124975)
  line L3 (-2.5, 1.124975) -> (-1.459131, 1.124975)
  line L4 (-1.5, 4.224976) -> (-1.5, 7.724976)
  line L5 (-1.5, 4.224976) -> (0, 4.224976)
  line L6 (0, 7.724976) -> (0, 4.224976)
  line L7 (-1.5, 7.724976) -> (0, 7.724976)
  line L8 (-1.5, 10.524974) -> (-1.5, 14.024974)
  line L9 (-1.5, 10.524974) -> (0, 10.524974)
  line L10 (0, 14.024974) -> (0, 10.524974)
  line L11 (-1.5, 14.024974) -> (0, 14.024974)
  line L12 (0.5, 3.724976) -> (-2, 3.724976)
  line L13 (-2, 3.724976) -> (-2, 8.224976)
  line L14 (-2, 8.224976) -> (0.5, 8.224976)
  line L15 (0.5, 8.224976) -> (0.5, 3.724976)
  line L16 (0.5, 10.024974) -> (-2, 10.024974)
  line L17 (-2, 10.024974) -> (-2, 14.524974)
  line L18 (-2, 14.524974) -> (0.5, 14.524974)
  line L19 (0.5, 14.524974) -> (0.5, 10.024974)
  line L20 (-1, 1.124975) -> (-2.5, 1.124975)
  line L21 (-1.459131, 1.124975) -> (-1, 1.124975)
  line L22 (-1, 1.124975) -> (-1, 17.624975)
  line L23 (-1, 17.624975) -> (-2.459131, 17.624975)
  line L24 (-2.459131, 17.624975) -> (-2.459131, 17.124975)
  line L25 (-2.5, 1.124975) -> (-2.5, 0.624975)
  line L26 (0, 0.624975) -> (-23.2, 0.624975)
  line L27 (-2.5, 0.624975) -> (0, 0.624975)
  line L28 (0, 0.624975) -> (0, 16.997106)
  line L29 (0, 65.920816) -> (0, 0.624975)
  line L30 (-2.459131, 17.624975) -> (-2.459131, 18.624975)
  line L31 (-2.447659, 18.624975) -> (0, 18.624975)
  arc A0 (-9.500816, 15.215286) -> (-4.410688, 30.505264) centre (-9.208398, 23.610194) ccw
  point P0 (23.709139, 15.26395)
  point P1 (-16.766975, 19.320809)
  point P2 (0, 3.724976)
  point P3 (-1, 3.724976)
  point P4 (0, 8.224976)
  point P5 (0, 10.024974)
  point P6 (-1, 10.024974)
  point P7 (-1, 8.224976)
  point P8 (-1, 14.524974)
  point P9 (0, 14.524974)
  point P10 (-2.459131, 18.609455)
  point P11 (-15.084098, 28.988231)
  point P12 (-1.575566, 19.478102)
  point P13 (-1.164182, 20.56642)
  point P14 (0, 14.524974)
  point P15 (0, 10.024974)
  point P16 (-1.459131, 8.224976)
  point P17 (-1.459131, 3.724976)
  point P18 (-9.516562, 14.590874)
  point P19 (-1.459131, 1.124975)
  point P20 (0, 14.024974)
  point P21 (0, 10.524974)
  dimension "d24" = 0.5
  dimension "d25" = 0.5
  dimension "d26" = 0.5
  dimension "d27" = 1
  constraints: 34 end point, 4 perpendicular, 4 point on line, 2 vertical, 1 collinear, 1 horizontal, 1 point on circle, 8 other
  measures "d24" distance between parallel lines of L5 L12
  measures "d25" distance between parallel lines of L9 L16
  measures "d26" distance between parallel lines of L1 L23
  measures "d27" distance between parallel lines of L23 L31
extrude "Extrusion7" add sketch "Sketch4" along normal blind 8 contours L22 L23 L30 A0 L31 L29 L28 L18 | L3 L20 L22 L12 L28 L26 L25 | L0 L12 L22 L20 | L16 L28 L14 L22
sketch "Sketch6" plane through (-23.709139, -10.164386, 14.531294) normal (0, 0.9970894, 0.0762418) x (1, 0, 0)
  circle A0 centre (-20.628356, 20.267276) radius 2.25
  circle A1 centre (-8.371644, 9.982674) radius 2.25
  point P0 (23.709139, 15.26395)
extrude "Extrusion8" cut sketch "Sketch6" against normal blind 2.6
sketch "Sketch7" plane through (-44.337494, -11.211604, -5.87522) normal (0, 0.9970894, 0.0762418) x (1, 0, 0)
  circle A0 centre (0, 0) radius 2.25
  circle A1 centre (12.256711, -10.284602) radius 2.25
  point P0 (44.337494, -5.003326)
hole "Hole2" at (-44.337494, -11.211604, -5.87522) at (-32.080783, -11.995721, 4.379447) direction (0, -0.9970894, -0.0762418) diameter 2.5 depth 10.6 counterbore diameter 4.5 counterbore depth 2.6
sketch "Sketch5" plane through (-23.709139, -14.311684, -51.899075) normal (0, 0.0762418, -0.9970894) x (-1, 0, 0)
  line L0 (23.2, 5.493888) -> (6.724879, 5.493888)
  line L1 (6, 9.993888) -> (6, 1.493888)
  circle A0 centre (16.7, 7.343888) radius 3.5
  circle A1 centre (9.5, 7.343888) radius 3.5
  point P0 (-23.709139, 18.226909)
  point P1 (23.2, 9.2)
  point P2 (5.901418, 4.6)
  point P3 (6.724879, 5.493888)
  dimension "d49" = 7
  dimension "d50" = 7
  dimension "d51" = 1.85
  dimension "d53" = 1.85
  constraints: 2 centre point, 2 end point, 1 tangent, 3 other
  measures "d49" diameter of A0
  measures "d50" diameter of A1
hole "Hole1" at (-40.409139, -6.989172, -51.339163) at (-33.209139, -6.989172, -51.339163) direction (0, -0.0762418, 0.9970894) diameter 2.459 depth 5 countersink diameter 3 countersink angle 90 thread size "M3x0.5" class "6H" standard "ISO Metric profile"
sketch "Sketch9" plane through (-13.003919, -14.919909, -24.270479) normal (0, 0.9970894, 0.0762418) x (-0.2526111, 0.0737692, -0.9647517)
  arc A0 (-15.739773, 17.703067) -> (-3.748905, 16.601338) centre (-9.208398, 22.985219) ccw
  point P0 (-25.59929, -6.756379)
  point P1 (-2.447659, 18)
  point P2 (-1.575566, 19.478102)
  point P3 (-9.500816, 14.590311)
  point P4 (-17.252614, 25.404018)
hole "Hole3" at (-32.917536, -16.04189, -9.597242) direction (0, -0.9970894, -0.0762418) diameter 2.5 depth 1.3
sketch "Sketch10" plane through (-23.709139, -10.164386, 14.531294) normal (0, 0.9970894, 0.0762418) x (1, 0, 0)
  line L0 (-23.2, 65.920816) -> (-23.2, 0.624975)
  circle A0 centre (-3.5, 61.795841) radius 3.5
  line L1 (0, 0.624975) -> (0, 65.920816)
  circle A1 centre (-19.2, 8.874975) radius 3.5
  circle A2 centre (-19.7, 47.525128) radius 3.5
  circle A3 centre (-3.392702, 45.015361) radius 3.5
  line L2 (-23.2, 5.374975) -> (-2.5, 5.374975)
  line L3 (-0.98734, 13.624975) -> (-23.2, 13.624975)
  circle A4 centre (-19.2, 8.874975) radius 2.5
  circle A5 centre (-19.971819, 24.971684) radius 3.5
  circle A6 centre (-19.971819, 24.971684) radius 2.5
  circle A7 centre (-20.628356, 20.267276) radius 2.25
  line L4 (-23.2, 0.624975) -> (-2.5, 0.624975)
  line L5 (0, 65.920816) -> (-23.2, 65.920816)
  line L6 (-2.5, 1.124975) -> (-2.5, 17.624975)
  line L7 (-1, 8.224976) -> (-1, 3.724976)
  line L8 (0, 18.624975) -> (0, 65.920816)
  line L9 (0, 14.524974) -> (-1, 14.524974)
  line L10 (-2.5, 0.624975) -> (-2.5, 1.124975)
  line L11 (0, 8.224976) -> (-1, 8.224976)
  line L12 (-1, 3.724976) -> (0, 3.724976)
  line L13 (0, 3.724976) -> (0, 8.224976)
  line L14 (-2.447659, 18.624975) -> (0, 18.624975)
  line L15 (-2.459131, 17.624975) -> (-2.459131, 18.609455)
  arc A8 (-9.500816, 15.215286) -> (-2.459131, 18.609455) centre (-9.208398, 23.610194) ccw
  arc A9 (-16.618436, 19.654018) -> (-9.500816, 15.215286) centre (-14.5, 15.124975) ccw
  arc A10 (-17.094606, 26.502896) -> (-16.618436, 19.654018) centre (-9.208398, 23.610194) ccw
  arc A11 (-4.410688, 30.505264) -> (-17.094606, 26.502896) centre (-13, 35.626174) ccw
  arc A12 (-2.447659, 18.624975) -> (-4.410688, 30.505264) centre (-9.208398, 23.610194) ccw
  line L16 (-1, 10.024974) -> (0, 10.024974)
  line L17 (0, 10.024974) -> (0, 14.524974)
  line L18 (-1, 14.524974) -> (-1, 10.024974)
  line L19 (-2.5, 17.624975) -> (-2.459131, 17.624975)
  point P0 (23.709139, 15.26395)
  dimension "d75" = 7
  dimension "d76" = 7
  dimension "d78" = 7
  dimension "d79" = 7
  dimension "d89" = 8.25
  dimension "d90" = 3.5
  dimension "d91" = 4.75
  dimension "d93" = 4
  dimension "d96" = 5
  dimension "d113" = 7
  dimension "d114" = 5
  dimension "d129" = 4.75
  constraints: 7 centre point, 4 end point, 3 tangent, 2 coincident, 2 point on line, 1 perpendicular
  measures "d75" diameter of A0
  measures "d76" diameter of A1
  measures "d78" diameter of A2
  measures "d79" diameter of A3
  measures "d89" distance between parallel lines of L3 L2
  measures "d90" distance from line of L2 A1.centre
  measures "d91" distance from line of L3 A1.centre
  measures "d93" distance from line of L0 A1.centre
  measures "d96" diameter of A4
  measures "d113" diameter of A5
  measures "d114" diameter of A6
  measures "d129" distance between parallel lines of L4 L2
hole "Hole4" at (-43.409139, -6.540983, -32.855506) at (-27.209139, -5.452957, -47.084681) at (-27.101841, -6.732332, -30.353043) at (-42.909139, -9.487742, 5.682151) at (-43.680957, -8.260499, -10.367707) direction (0, -0.9970894, -0.0762418) diameter 4 depth 3 counterbore diameter 4.5 counterbore depth 0.5
sketch "Sketch11" plane through (-46.909139, -15.94337, -30.559913) normal (-1, 0, 0) x (0, -0.0762418, 0.9970894)
  line L0 (-21.401454, 9.2) -> (43.894386, 9.2)
  line L1 (34.269362, 9.2) -> (34.269362, 0)
  line L2 (43.894386, 0) -> (-0.624975, 0)
  line L3 (27.127061, 9.2) -> (27.127061, 0)
  line L4 (34.269362, 9.2) -> (27.127061, 0)
  line L5 (27.127061, 9.2) -> (34.269362, 0)
  line L6 (20.127061, 9.2) -> (20.127061, 0)
  line L7 (-6.73983, 2.1) -> (-6.73983, 9.2)
  line L8 (43.894386, 9.2) -> (-21.401454, 9.2)
  circle A0 centre (-11.956561, 4.6) radius 2.5
  line L9 (-2.425932, 2.1) -> (-0.624975, 2.1)
  circle A1 centre (20.127061, 3) radius 2.5
  point P0 (29.255412, 18.226909)
  point P1 (27.127061, 5.4)
  point P2 (22.627061, 5.4)
  point P3 (34.269362, 6.199888)
  point P4 (44.519362, 5.899888)
  point P5 (0, 0)
  point P6 (30.698211, 4.6)
  point P7 (18.016466, 9.2)
  point P8 (25.894386, 9.2)
  point P9 (14.014098, 9.2)
  point P10 (41.129565, 9.193888)
  point P11 (-21.401454, 0)
  point P12 (-21.401454, 2.093888)
  point P13 (43.894386, 9.2)
  point P14 (29.304076, 9.2)
  dimension "d98" = 5
  dimension "d115" = 5
  dimension "d116" = 0.5
  dimension "d117" = 7
  dimension "d130" = 5.21673
  constraints: 12 end point, 6 point on line, 2 centre point, 2 perpendicular, 2 vertical, 1 midpoint, 9 other
  measures "d98" diameter of A0
  measures "d115" diameter of A1
  measures "d116" distance edge to line of A1 L2
  measures "d117" distance between parallel lines of L3 L6
  measures "d130" distance from line of L7 A0.centre
hole "Hole5" at (-46.909139, -13.697247, 0.399659) at (-46.909139, -10.445169, -42.130959) at (-46.909139, -14.486626, -10.262709) direction (1, 0, 0) diameter 4 depth 3.5 counterbore diameter 4.5 counterbore depth 0.5
body "Solid2"
